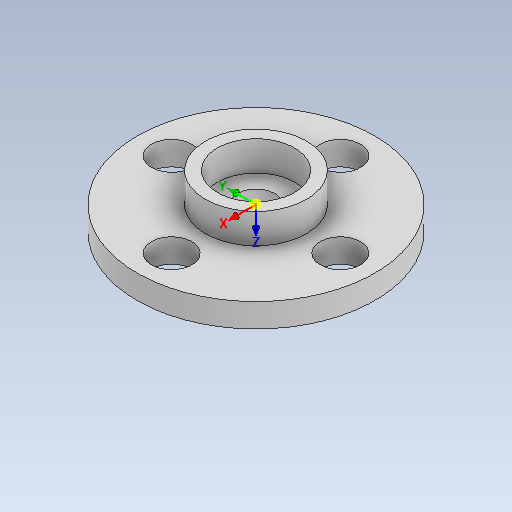
# Autodesk Inventor part: Servo krepej
Saved by Autodesk Inventor 2020 (Build 240168000, 168)
## iProperties
Created: 2020-01-16
Part Number: Servo krepej
Material: Типовые
Document SubType Name: Modeling
Designer: Windows
Density: 1 g/cm^3
Appearance: По умолчанию
Author: Windows
Autodesk Inventor part; units mm, degrees
ref_plane "YZ Plane" through (0, 0, 0) normal (1, 0, 0) x (0, 1, 0)
ref_plane "XZ Plane" through (0, 0, 0) normal (0, 1, 0) x (-1, 0, 0)
ref_plane "XY Plane" through (0, 0, 0) normal (0, 0, 1) x (1, 0, 0)
sketch "Эскиз1" plane through (0, 0, 0) normal (0, 1, 0) x (-1, 0, 0)
  circle A0 centre (0, 0) radius 10
  circle A1 centre (0, 0) radius 1.6
  circle A2 centre (0, 7.1) radius 1.7
  circle A3 centre (-7.1, 0) radius 1.7
  circle A4 centre (0, -7.1) radius 1.7
  circle A5 centre (7.1, 0) radius 1.7
  dimension "d0" = 20
  dimension "d1" = 3.2
  dimension "d2" = 3.4
  dimension "d3" = 1.2
  dimension "d6" = 360
  constraints: 6 centre point, 2 coincident, 9 other
  measures "d0" diameter of A0
  measures "d1" diameter of A1
  measures "d2" diameter of A2
extrude "Выдавливание1" add sketch "Эскиз1" along normal blind 2
sketch "Эскиз2" plane through (0, 2, 0) normal (0, 1, 0) x (1, 0, 0)
  circle A0 centre (0, 0) radius 1.6 projected
  circle A1 centre (0, 0) radius 4.25
  circle A2 centre (0, 0) radius 3.25
  dimension "d10" = 8.5
  dimension "d11" = 6.5
  constraints: 2 centre point, 2 coincident
  measures "d10" diameter of A1
  measures "d11" diameter of A2
extrude "Выдавливание2" add sketch "Эскиз2" along normal blind 2.5 contours A1
